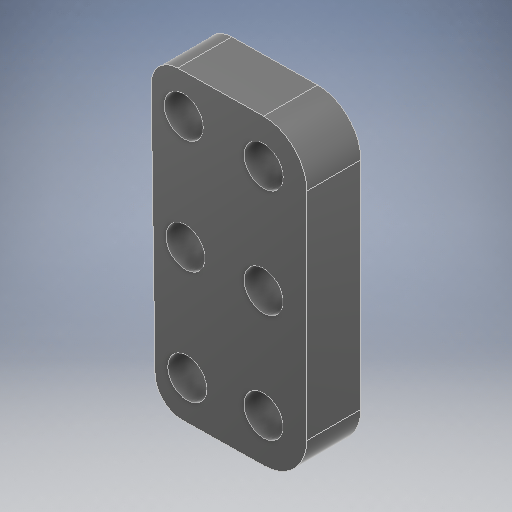
# Autodesk Inventor part: OdomPods
Saved by Autodesk Inventor 2026.1 (Build 301233000, 233)
## iProperties
Created: 2025-10-06
Part Number: OdomPods
Material: Plastic, Opaque Black
Document SubType Name: Modeling
Designer: Teddy
Density: 0.952 g/cm^3
Appearance: Smooth - Black
Author: Teddy
Autodesk Inventor part; units mm, degrees
ref_plane "YZ Plane" through (0, 0, 0) normal (1, 0, 0) x (0, 1, 0)
ref_plane "XZ Plane" through (0, 0, 0) normal (0, 1, 0) x (-1, 0, 0)
ref_plane "Work Plane1" through (0.394452, -0.667998, 0) normal (0, 0, 1) x (0.9998788, 0.0155691, 0)
sketch "Sketch1" plane through (0.394452, -0.667998, 0) normal (0, 0, 1) x (0.9998788, 0.0155691, 0)
  circle A0 centre (5.204347, 38.285312) radius 1.27
  circle A1 centre (5.004519, 25.586884) radius 1.27
  circle A2 centre (4.796193, 12.888588) radius 1.27
  line L0 (5.002396, 38.285413) -> (4.989697, 12.888491) construction
  line L1 (0.125003, 38.366943) -> (-0.283151, 12.970219)
  line L2 (9.875538, 12.806957) -> (10.283691, 38.203681)
  arc A3 (10.283691, 38.203681) -> (0.125003, 38.366943) centre (5.204347, 38.285312) ccw
  arc A4 (-0.283151, 12.970219) -> (9.875538, 12.806957) centre (4.796193, 12.888588) ccw
  circle A5 centre (4.796193, 12.888588) radius 2.286
  circle A6 centre (4.996047, 25.587018) radius 2.286
  circle A7 centre (5.204347, 38.285312) radius 2.286
  line L3 (4.714563, 7.809244) -> (-4.810437, 7.809244)
  line L4 (-7.985437, 10.984244) -> (-7.985437, 40.194244)
  line L5 (-4.808994, 43.369244) -> (5.285978, 43.364656)
  arc A8 (-7.985437, 10.984244) -> (-4.810437, 7.809244) centre (-4.810437, 10.984244) ccw
  arc A9 (-4.808994, 43.369244) -> (-7.985437, 40.194244) centre (-4.810437, 40.194244) ccw
  circle A10 centre (-4.175437, 12.381244) radius 2.286
  circle A11 centre (-4.175437, 25.586884) radius 2.286
  circle A12 centre (-4.175437, 38.796956) radius 2.286
  point P0 (-0.384004, 0.674059)
  point P1 (-7.985437, 7.809244)
  dimension "d0" = 10.16
  dimension "d1" = 4.572
  dimension "d2" = 4.572
  dimension "d3" = 4.572
  dimension "d4" = 12.7
  dimension "d6" = 3.175
  dimension "d7" = 3.175
  dimension "d8" = 35.56
  dimension "d18" = 3.81
  dimension "d19" = 4.572
  dimension "d20" = 4.572
  dimension "d21" = 4.572
  constraints: 14 end point, 10 centre point, 10 point on circle, 8 tangent, 3 coincident, 3 point on line, 2 equal radius, 2 vertical alignment, 1 horizontal, 1 horizontal alignment, 1 parallel, 1 perpendicular, 1 other
  measures "d0" diameter of A4
  measures "d1" diameter of A5
  measures "d2" diameter of A6
  measures "d3" diameter of A7
  measures "d4" distance of L3.start point (-7.985, 7.809)
  measures "d6" radius of A8
  measures "d7" radius of A9
  measures "d8" distance of L5.start L3.end
  measures "d18" distance from line of L4 A10.centre
  measures "d19" diameter of A10
  measures "d20" distance from line of L3 A10.centre
  measures "d21" distance from line of L5 A12.centre
sketch "Sketch1 outline for Extrusion1" plane through (0.394452, -0.667998, 0) normal (0, 0, 1) x (0.9998788, 0.0155691, 0)
  line L0 (5.285978, 43.364656) -> (-4.808994, 43.369244)
  arc A0 (10.283691, 38.203681) -> (5.285978, 43.364656) centre (5.204347, 38.285312) ccw
  arc A1 (-4.808994, 43.369244) -> (-7.985437, 40.194244) centre (-4.810437, 40.194244) ccw
  line L1 (9.875538, 12.806957) -> (10.283691, 38.203681)
  line L2 (-7.985437, 40.194244) -> (-7.985437, 10.984244)
  arc A2 (4.714563, 7.809244) -> (9.875538, 12.806957) centre (4.796193, 12.888588) ccw
  arc A3 (-7.985437, 10.984244) -> (-4.810437, 7.809244) centre (-4.810437, 10.984244) ccw
  line L3 (-4.810437, 7.809244) -> (4.714563, 7.809244)
  circle A4 centre (-4.175437, 12.381244) radius 2.286
  circle A5 centre (-4.175437, 25.586884) radius 2.286
  circle A6 centre (4.796193, 12.888588) radius 2.286
  circle A7 centre (4.996047, 25.587018) radius 2.286
  circle A8 centre (-4.175437, 38.796956) radius 2.286
  circle A9 centre (5.204347, 38.285312) radius 2.286
extrude "Extrusion1" add sketch "Sketch1 outline for Extrusion1" along normal blind 6.35
body "Solid1"
